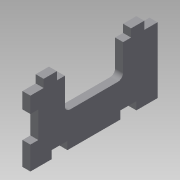
# Autodesk Inventor part: TerminalPlate
Saved by Autodesk Inventor 2013 (Build 170138000, 138)
## iProperties
Created: 2013-12-12
Part Number: TerminalPlate
Material: Generic
Document SubType Name: Modeling
Designer: Eric
Density: 1 g/cm^3
Author: Eric
Autodesk Inventor part; units mm, degrees
ref_plane "YZ Plane" through (0, 0, 0) normal (1, 0, 0) x (0, 1, 0)
ref_plane "XZ Plane" through (0, 0, 0) normal (0, 1, 0) x (-1, 0, 0)
ref_plane "XY Plane" through (0, 0, 0) normal (0, 0, 1) x (1, 0, 0)
sketch "Sketch1" plane through (0, 0, 0) normal (1, 0, 0) x (0, 1, 0)
  line L0 (0, 15.7949) -> (-3, 15.7949)
  line L1 (-3, 5.7949) -> (0, 5.7949)
  line L2 (10, 21.7949) -> (10, 11.7949)
  line L3 (12, 9.7949) -> (30, 9.7949)
  line L4 (35, 21.7949) -> (32, 21.7949)
  line L5 (32, 21.7949) -> (32, 11.7949)
  line L6 (7, 21.7949) -> (10, 21.7949)
  line L7 (2, 21.7949) -> (2, 24.7949)
  line L8 (2, 24.7949) -> (7, 24.7949)
  line L9 (7, 24.7949) -> (7, 21.7949)
  line L10 (35, 21.7949) -> (35, 24.7949)
  line L11 (35, 24.7949) -> (40, 24.7949)
  line L12 (40, 24.7949) -> (40, 21.7949)
  line L13 (-3, 15.7949) -> (-3, 21.7949)
  line L14 (45, -3) -> (45, 21.7949)
  line L15 (40, 21.7949) -> (45, 21.7949)
  line L16 (2, 21.7949) -> (-3, 21.7949)
  line L17 (0, 5.7949) -> (0, 15.7949)
  arc A0 (10, 11.7949) -> (12, 9.7949) centre (12, 11.7949) ccw
  arc A1 (30, 9.7949) -> (32, 11.7949) centre (30, 11.7949) ccw
  line L18 (5, 0) -> (5, -3)
  line L19 (5, -3) -> (-3, -3)
  line L20 (-3, 5.7949) -> (-3, -3)
  line L21 (5, 0) -> (11, 0)
  line L22 (11, 0) -> (11, -3)
  line L23 (11, -3) -> (31, -3)
  line L24 (31, -3) -> (31, 0)
  line L25 (31, 0) -> (37, 0)
  line L26 (37, 0) -> (37, -3)
  line L27 (37, -3) -> (45, -3)
  point P0 (0, 0)
  point P1 (32, 9.7949)
  point P2 (10, 9.7949)
  dimension "d6" = 3
  dimension "d7" = 3
  dimension "d8" = 10
  dimension "d70" = 5
  dimension "d71" = 3
  dimension "d72" = 5
  dimension "d74" = 2
  dimension "d75" = 5
  dimension "d76" = 5
  dimension "d78" = 48
  dimension "d79" = 13
  dimension "d80" = 13
  dimension "d83" = 3
  dimension "d86" = 6
  dimension "d88" = 8
  dimension "d89" = 6
  dimension "d90" = 6
  dimension "d91" = 8
  dimension "d92" = 3
  dimension "d93" = 3
  constraints: 56 end point, 9 parallel, 8 perpendicular, 6 horizontal alignment, 5 horizontal, 4 point on circle, 4 point on line, 4 tangent, 2 centre point, 2 collinear, 1 equal radius
  measures "d6" distance of L0.start L0.end
  measures "d7" distance of L1.start L1.end
  measures "d8" distance of L0.end L1.start
  measures "d70" distance of L7.end L8.end
  measures "d71" distance of L11.end L12.end
  measures "d72" distance of L10.end L11.end
  measures "d74" radius of A0
  measures "d75" distance between parallel lines of L14 L12
  measures "d76" distance between parallel lines of L13 L7
  measures "d78" distance between parallel lines of L13 L14
  measures "d79" distance between parallel lines of L13 L2
  measures "d80" distance between parallel lines of L14 L5
  measures "d83" distance of L7.start L7.end
  measures "d86" distance of L0.end L13.end
  measures "d88" distance of L18.end L19.end
  measures "d89" distance of L18.start L21.end
  measures "d90" distance of L24.end L25.end
  measures "d91" distance of L26.end L14.start
  measures "d92" distance of L18.start L18.end
  measures "d93" distance of L25.end L26.end
extrude "Extrusion1" add sketch "Sketch1" along normal blind 3
body "Solid1"
